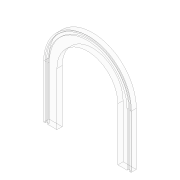
# Autodesk Inventor part: Tapa Frontar y Posterior
Saved by Autodesk Inventor 2022 (Build 260153000, 153)
## iProperties
Created: 2021-08-17
Part Number: Tapa Frontar y Posterior
Material: Acrylic
Document SubType Name: Modeling
Designer: cristiano.schuster
Density: 1.188 g/cm^3
Appearance: Transparent - Clear
Author: cristiano.schuster
Autodesk Inventor part; units mm, degrees
ref_plane "YZ Plane" through (0, 0, 0) normal (1, 0, 0) x (0, 1, 0)
ref_plane "XZ Plane" through (0, 0, 0) normal (0, 1, 0) x (-1, 0, 0)
ref_plane "XY Plane" through (0, 0, 0) normal (0, 0, 1) x (1, 0, 0)
sketch "Sketch1" plane through (0, 0, 0) normal (0, 0, 1) x (1, 0, 0)
  arc A0 (82.5, 0) -> (-82.5, 0) centre (0, 0) ccw
  line L0 (-82.5, 0) -> (-82.5, -100)
  line L1 (82.5, 0) -> (82.5, -100)
  arc A1 (-82.5, 0) -> (82.5, 0) centre (0, 0) ccw construction
  arc A2 (57.5, 0) -> (-57.5, 0) centre (0, 0) ccw
  line L2 (-57.5, 0) -> (-57.5, -100)
  line L3 (-57.5, -100) -> (-82.5, -100)
  line L4 (82.5, -100) -> (57.5, -100)
  line L5 (57.5, -100) -> (57.5, 0)
  arc A3 (-57.5, 0) -> (57.5, 0) centre (0, 0) ccw construction
  dimension "d0" = 165
  dimension "d1" = 100
  dimension "d2" = 100
  dimension "d4" = 115
  constraints: 12 end point, 8 point on circle, 4 centre point, 4 tangent, 4 vertical, 2 coincident, 1 perpendicular, 1 point on line
  measures "d0" diameter of A0
  measures "d1" vertical distance of L0.end point (0, 0)
  measures "d2" distance of L1.start L1.end
  measures "d4" diameter of A2
extrude "Extrusion1" add sketch "Sketch1" along normal blind 10
sketch "Sketch2" plane through (0, 0, 10) normal (0, 0, 1) x (1, 0, 0)
  arc A0 (80, 0) -> (-80, 0) centre (0, 0) ccw
  arc A1 (75, 0) -> (-75, 0) centre (0, 0) ccw
  line L0 (-80, 0) -> (-80, -100)
  line L1 (-82.5, -100) -> (-57.5, -100) projected
  line L2 (-75, 0) -> (-75, -100)
  line L3 (75, 0) -> (75, -100)
  line L4 (57.5, -100) -> (82.5, -100) projected
  line L5 (80, 0) -> (80, -100)
  dimension "d7" = 160
  dimension "d8" = 150
  constraints: 8 end point, 4 point on circle, 3 horizontal alignment, 3 point on line, 3 vertical, 2 centre point, 2 coincident, 1 parallel, 1 tangent
  measures "d7" diameter of A0
  measures "d8" diameter of A1
extrude "Extrusion2" cut sketch "Sketch2" against normal blind 3
body "Solid1"
